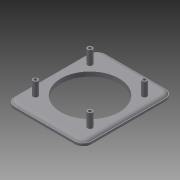
# Autodesk Inventor part: Speaker Front Plate
Saved by Autodesk Inventor 2014 SP2 (Build 180246200, 246)
## iProperties
Created: 2015-08-12
Part Number: Speaker Front Plate
Material: Generic
Document SubType Name: Modeling
Designer: Devon
Density: 1 g/cm^3
Appearance: Default
Author: Devon
Autodesk Inventor part; units mm, degrees
ref_plane "YZ Plane" through (0, 0, 0) normal (1, 0, 0) x (0, 1, 0)
ref_plane "XZ Plane" through (0, 0, 0) normal (0, 1, 0) x (-1, 0, 0)
ref_plane "XY Plane" through (0, 0, 0) normal (0, 0, 1) x (1, 0, 0)
sketch "Sketch1" plane through (0, 0, 0) normal (0, 1, 0) x (-1, 0, 0)
  circle A0 centre (0, 0) radius 22.6568
  line L0 (0, 35.306) -> (23.5585, 35.306)
  line L1 (29.9085, 28.956) -> (29.9085, -28.956)
  line L2 (23.5585, -35.306) -> (-23.5585, -35.306)
  line L3 (-29.9085, -28.956) -> (-29.9085, 28.956)
  line L4 (-23.5585, 35.306) -> (0, 35.306)
  arc A1 (29.9085, 28.956) -> (23.5585, 35.306) centre (23.5585, 28.956) ccw
  arc A2 (23.5585, -35.306) -> (29.9085, -28.956) centre (23.5585, -28.956) ccw
  arc A3 (-29.9085, -28.956) -> (-23.5585, -35.306) centre (-23.5585, -28.956) ccw
  arc A4 (-23.5585, 35.306) -> (-29.9085, 28.956) centre (-23.5585, 28.956) ccw
  point P0 (29.9085, 35.306)
  point P1 (29.9085, -35.306)
  point P2 (-29.9085, -35.306)
  dimension "d0" = 45.3136
  dimension "d1" = 35.306
  dimension "d2" = 29.9085
  dimension "d3" = 70.612
  dimension "d4" = 59.817
  dimension "d5" = 6.35
  constraints: 10 end point, 8 point on circle, 8 tangent, 6 point on line, 5 centre point, 3 equal radius, 3 perpendicular, 1 coincident, 1 parallel
  measures "d0" diameter of A0
  measures "d1" distance of A0.centre L0.start
  measures "d2" distance of L0.start point (29.909, 35.306)
  measures "d3" distance of point (29.909, 35.306) point (29.909, -35.306)
  measures "d4" distance of point (29.909, -35.306) point (-29.909, -35.306)
  measures "d5" radius of A1
extrude "Extrusion1" add sketch "Sketch1" along normal blind 1.778
sketch "Sketch2" plane through (0, 1.778, 0) normal (0, 1, 0) x (1, 0, 0)
  circle A0 centre (0, 0) radius 22.6568 projected
  line L0 (-23.5585, -35.306) -> (23.5585, -35.306) projected
  line L1 (29.9085, -28.956) -> (29.9085, 28.956) projected
  line L2 (23.5585, 35.306) -> (-23.5585, 35.306) projected
  line L3 (-29.9085, 28.956) -> (-29.9085, -28.956) projected
  line L4 (0, 35.306) -> (0, 34.671)
  line L5 (29.9085, 0) -> (29.2735, 0)
  line L6 (0, -35.306) -> (0, -34.671)
  line L7 (-29.9085, 0) -> (-29.2735, 0)
  line L8 (0, 34.671) -> (-23.5585, 34.671)
  line L9 (-29.2735, 28.956) -> (-29.2735, 0)
  line L10 (0, 34.671) -> (23.5585, 34.671)
  line L11 (29.2735, 28.956) -> (29.2735, 0)
  line L12 (0, -34.671) -> (23.5585, -34.671)
  line L13 (29.2735, -28.956) -> (29.2735, 0)
  line L14 (0, -34.671) -> (-23.5585, -34.671)
  line L15 (-29.2735, -28.956) -> (-29.2735, 0)
  arc A1 (23.5585, -34.671) -> (29.2735, -28.956) centre (23.5585, -28.956) ccw
  arc A2 (29.2735, 28.956) -> (23.5585, 34.671) centre (23.5585, 28.956) ccw
  arc A3 (-23.5585, 34.671) -> (-29.2735, 28.956) centre (-23.5585, 28.956) ccw
  arc A4 (-29.2735, -28.956) -> (-23.5585, -34.671) centre (-23.5585, -28.956) ccw
  circle A5 centre (0, 0) radius 22.6568
  dimension "d8" = 0.635
  dimension "d9" = 0.635
  dimension "d10" = 0.635
  dimension "d11" = 0.635
  dimension "d12" = 5.715
  constraints: 24 end point, 8 point on circle, 8 tangent, 5 centre point, 5 perpendicular, 4 equal radius, 4 midpoint, 2 horizontal, 1 coincident, 1 parallel
  measures "d8" distance of L4.start L4.end
  measures "d9" distance of L5.start L5.end
  measures "d10" distance of L6.start L6.end
  measures "d11" distance of L7.start L7.end
  measures "d12" radius of A1
extrude "Extrusion2" add sketch "Sketch2" along normal blind 1.651
fillet "Fillet1" radius 3.175 8 edges at (27.5996, 3.429, -32.9971) (0, 3.429, -34.671) (-27.5996, 3.429, -32.9971) (-29.2735, 3.429, 0) (-27.5996, 3.429, 32.9971) (0, 3.429, 34.671) (27.5996, 3.429, 32.9971) (29.2735, 3.429, 0)
sketch "Sketch3" plane through (0, 3.429, 0) normal (0, 1, 0) x (1, 0, 0)
  circle A0 centre (0, 0) radius 22.6568 projected
  circle A1 centre (0, 0) radius 25.146
  line L0 (-26.2636, 0) -> (-25.5008, 22.4355)
  line L1 (-22.4355, 25.5008) -> (0, 26.2636)
  line L2 (0, 26.2636) -> (22.4355, 25.5008)
  line L3 (25.5008, 22.4355) -> (26.2636, 0)
  line L4 (26.2636, 0) -> (25.5008, -22.4355)
  line L5 (22.4355, -25.5008) -> (0, -26.2636)
  line L6 (0, -26.2636) -> (-22.4355, -25.5008)
  line L7 (-25.5008, -22.4355) -> (-26.2636, 0)
  arc A2 (25.5008, 22.4355) -> (22.4355, 25.5008) centre (22.3276, 22.3276) ccw
  arc A3 (22.4355, -25.5008) -> (25.5008, -22.4355) centre (22.3276, -22.3276) ccw
  arc A4 (-25.5008, -22.4355) -> (-22.4355, -25.5008) centre (-22.3276, -22.3276) ccw
  arc A5 (-22.4355, 25.5008) -> (-25.5008, 22.4355) centre (-22.3276, 22.3276) ccw
  circle A6 centre (-21.1768, 21.1768) radius 1.9812
  circle A7 centre (-21.1768, 21.1768) radius 1.143
  circle A8 centre (21.1768, 21.1768) radius 1.9812
  circle A9 centre (21.1768, 21.1768) radius 1.143
  circle A10 centre (21.1768, -21.1768) radius 1.9812
  circle A11 centre (21.1768, -21.1768) radius 1.143
  circle A12 centre (-21.1768, -21.1768) radius 1.9812
  circle A13 centre (-21.1768, -21.1768) radius 1.143
  point P0 (25.4, 25.4)
  point P1 (-25.4, -25.4)
  point P2 (-25.4, 25.4)
  point P3 (25.4, -25.4)
  dimension "d20" = 50.8
  dimension "d36" = 50.292
  dimension "d39" = 50.8
  dimension "d40" = 50.8
  dimension "d41" = 50.8
  dimension "d46" = 3.175
  dimension "d47" = 3.9624
  dimension "d48" = 2.286
  dimension "d49" = 3.9624
  dimension "d50" = 2.286
  dimension "d51" = 3.9624
  dimension "d52" = 2.286
  dimension "d53" = 3.9624
  dimension "d54" = 2.286
  constraints: 16 end point, 13 centre point, 8 point on circle, 8 point on line, 8 tangent, 5 coincident, 3 equal radius
  measures "d20" distance of point (-25.4, -25.4) point (-25.4, 25.4)
  measures "d36" diameter of A1
  measures "d39" distance of point (25.4, 25.4) point (25.4, -25.4)
  measures "d40" distance of point (25.4, -25.4) point (-25.4, -25.4)
  measures "d41" distance of point (-25.4, -25.4) point (-25.4, 25.4)
  measures "d46" radius of A2
  measures "d47" diameter of A6
  measures "d48" diameter of A7
  measures "d49" diameter of A8
  measures "d50" diameter of A9
  measures "d51" diameter of A10
  measures "d52" diameter of A11
  measures "d53" diameter of A12
  measures "d54" diameter of A13
extrude "Extrusion4" add sketch "Sketch3" along normal blind 10.6172 contours A6 | A8 | A10 | A12
body "Solid1"
